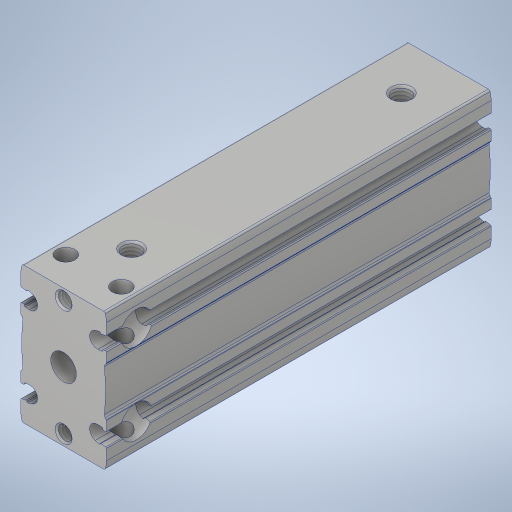
# Autodesk Inventor part: 4186566 DPDM-50---(h)
Saved by Autodesk Inventor 2024 (Build 280153000, 153)
## iProperties
Created: 2024-04-11
Part Number: 4186566 DPDM-50---(h)
Material: Aluminum 6061
Catalog Web Link: www.cadenas.de
Description: DPDM(h)-housing
Vendor: FESTO
Document SubType Name: Modeling
Designer: psAdmin
Manufacturer: FESTO
Mass: 104.929 g
Surface Area: 178.452 cm^2
Volume: 38.8626 cm^3
Density: 2.7 g/cm^3
Appearance: Aluminum - Flat
Category: PARTsolutions
Company: FESTO
PSOL_IDENT_0: {$CADENAS_DATA/23d-libs/festo/parts/d/dpdm/parts/dpdm_housing.prj},201 {VTYP=3D},{NB=4186566 DPDM-50
PSOL_IDENT_1: ---(h)},{LINA=4186566 DPDM-50---(h)},{NN=DPDM(h)},{DATE=23.02.2024 06:49:52},{GEOMDATE=23.02.2024 06
PSOL_IDENT_2: :49:00},{VERSION=},{LINEID=30},{WBVAR=VER,HUB,FUN,KOT},{WBNUMERIC=HUB}  {NB=4186566 DPDM-50---(h)},{
PSOL_IDENT_3: LINA=4186566 DPDM-50---(h)},{KT=DUMMY},{TNR=4186566},{TYP=DPDM},{VER=-},{VERNB=},{KOL=16},{HUB=50},{
PSOL_IDENT_4: HUB1=5,10,15,20,25,30,40,50},{FUN=-},{FUN1='-'},{FUNNB=},{KOT=-},{KOT1='-','H','T'},{KOTNB=},{MM=6.0
PSOL_IDENT_5: 00},{L2=40.000},{EE=M5},{EEN=5.000},{ET=4.500},{BG=6.000},{RT=M4},{RTN=4.000},{H2=19.000},{E=20.000}
PSOL_IDENT_6: ,{UO=32.000},{TO=27.000},{H3=13.000},{LX=7.000},{PL=24.100},{PR=11.000},{U1=0.000},{D5=4.300},{D6=7.
PSOL_IDENT_7: 500},{T1=6.000},{A1X=6.000},{A1Y=2.000},{A2X=6.100},{A2Y=9.100},{W2=10.000},{R1=47.500},{A3=11.500},
PSOL_IDENT_8: {L1=22.6},{L3=7.000},{DQ=4.000}
NB: 4186566 DPDM-50---(h)
NN: DPDM(h)
NT: housing
NBSYN: $TNR. $TYP.$VERNB.-$HUB.$FUNNB.$KOTNB.---(h)
LINA: 4186566 DPDM-50---(h)
CATALOG: Festo
TNR: 4186566
TYP: DPDM
VER: -
KOL: 16
HUB: 50
FUN: -
KOT: -
MM: 6
L2: 40
EE: M5
EEN: 5
ET: 4.5
BG: 6
RT: M4
RTN: 4
H2: 19
E: 20
UO: 32
TO: 27
H3: 13
LX: 7
PL: 24.1
PR: 11
U1: 0
D5: 4.3
D6: 7.5
T1: 6
A1X: 6
A1Y: 2
A2X: 6.1
A2Y: 9.1
W2: 10
R1: 47.5
A3: 11.5
L3: 7
DQ: 4
SUPPLIER: FESTO
ARTICLENO: 4186566 DPDM-50---(h)
BOMINFO: 4186566 DPDM-50---(h)
CREATOR: CADENAS GmbH
Title: 4186566 DPDM-50---(h)
Author: Cadenas PARTsolutions
Comments: housing
Autodesk Inventor part; units mm, degrees
sketch "Sketch_1" plane through (0, 0, 0) normal (0, 0, 1) x (1, 0, 0)
  line L0 (-10, -16) -> (10, -16)
  line L1 (10, -16) -> (10, 16)
  line L2 (10, 16) -> (-10, 16)
  line L3 (-10, 16) -> (-10, -16)
  constraints: 8 end point
extrude "Extrusion1" add sketch "Sketch_1" against normal blind 90
sketch "Sketch_2" plane through (0, 0, 0) normal (0, 0, 1) x (1, 0, 0)
  line L0 (-20, -26) -> (20, -26)
  line L1 (20, -26) -> (20, 26)
  line L2 (20, 26) -> (-20, 26)
  line L3 (-20, 26) -> (-20, -26)
  line L4 (-10, 8.0262) -> (-10, -8.0262)
  arc A0 (-10, -8.0262) -> (-9.7653, -8.2231) centre (-9.8, -8.0262) ccw
  line L5 (-9.7653, -8.2231) -> (-9.2952, -8.1403)
  arc A1 (-9.2952, -8.1403) -> (-9.1492, -7.9314) centre (-9.3265, -7.963) ccw
  arc A2 (-8.9688, -7.697) -> (-9.1492, -7.9314) centre (-8.9523, -7.8963) ccw
  line L6 (-8.9688, -7.697) -> (-8.0209, -7.6187)
  arc A3 (-7.3984, -11.149) -> (-8.0209, -7.6187) centre (-7.8727, -9.4126) ccw
  line L7 (-7.3984, -11.149) -> (-8.316, -11.3996)
  arc A4 (-8.5657, -11.241) -> (-8.316, -11.3996) centre (-8.3687, -11.2066) ccw
  arc A5 (-8.5657, -11.241) -> (-8.7743, -11.0947) centre (-8.743, -11.2719) ccw
  line L8 (-8.7743, -11.0947) -> (-9.8347, -11.2817)
  arc A6 (-9.8347, -11.2817) -> (-10, -11.4786) centre (-9.8, -11.4786) ccw
  line L9 (-10, -11.4786) -> (-10, -14)
  arc A7 (-10, -14) -> (-9.7564, -15.6923) centre (-4, -14) ccw
  arc A8 (-9.7564, -15.6923) -> (-9.3452, -16) centre (-9.3452, -15.5714) ccw
  line L10 (-9.3452, -16) -> (9.3452, -16)
  arc A9 (9.3452, -16) -> (9.7564, -15.6923) centre (9.3452, -15.5714) ccw
  arc A10 (9.7564, -15.6923) -> (10, -14) centre (4, -14) ccw
  line L11 (10, -14) -> (10, -11.4786)
  arc A11 (10, -11.4786) -> (9.8347, -11.2817) centre (9.8, -11.4786) ccw
  line L12 (9.8347, -11.2817) -> (8.7743, -11.0947)
  arc A12 (8.7743, -11.0947) -> (8.5657, -11.241) centre (8.743, -11.2719) ccw
  arc A13 (8.316, -11.3996) -> (8.5657, -11.241) centre (8.3687, -11.2066) ccw
  line L13 (8.316, -11.3996) -> (7.3984, -11.149)
  arc A14 (8.0209, -7.6187) -> (7.3984, -11.149) centre (7.8727, -9.4126) ccw
  line L14 (8.0209, -7.6187) -> (8.9688, -7.697)
  arc A15 (9.1492, -7.9314) -> (8.9688, -7.697) centre (8.9523, -7.8963) ccw
  arc A16 (9.1492, -7.9314) -> (9.2952, -8.1403) centre (9.3265, -7.963) ccw
  line L15 (9.2952, -8.1403) -> (9.7653, -8.2231)
  arc A17 (9.7653, -8.2231) -> (10, -8.0262) centre (9.8, -8.0262) ccw
  line L16 (10, -8.0262) -> (10, 8.0262)
  arc A18 (10, 8.0262) -> (9.7653, 8.2231) centre (9.8, 8.0262) ccw
  line L17 (9.7653, 8.2231) -> (9.2952, 8.1403)
  arc A19 (9.2952, 8.1403) -> (9.1492, 7.9314) centre (9.3265, 7.963) ccw
  arc A20 (8.9688, 7.697) -> (9.1492, 7.9314) centre (8.9523, 7.8963) ccw
  line L18 (8.9688, 7.697) -> (8.0209, 7.6187)
  arc A21 (7.3984, 11.149) -> (8.0209, 7.6187) centre (7.8727, 9.4126) ccw
  line L19 (7.3984, 11.149) -> (8.316, 11.3996)
  arc A22 (8.5657, 11.241) -> (8.316, 11.3996) centre (8.3687, 11.2066) ccw
  arc A23 (8.5657, 11.241) -> (8.7743, 11.0947) centre (8.743, 11.2719) ccw
  line L20 (8.7743, 11.0947) -> (9.8347, 11.2817)
  arc A24 (9.8347, 11.2817) -> (10, 11.4786) centre (9.8, 11.4786) ccw
  line L21 (10, 11.4786) -> (10, 14)
  arc A25 (10, 14) -> (9.7564, 15.6923) centre (4, 14) ccw
  arc A26 (9.7564, 15.6923) -> (9.3452, 16) centre (9.3452, 15.5714) ccw
  line L22 (9.3452, 16) -> (-9.3452, 16)
  arc A27 (-9.3452, 16) -> (-9.7564, 15.6923) centre (-9.3452, 15.5714) ccw
  arc A28 (-9.7564, 15.6923) -> (-10, 14) centre (-4, 14) ccw
  line L23 (-10, 14) -> (-10, 11.4786)
  arc A29 (-10, 11.4786) -> (-9.8347, 11.2817) centre (-9.8, 11.4786) ccw
  line L24 (-9.8347, 11.2817) -> (-8.7743, 11.0947)
  arc A30 (-8.7743, 11.0947) -> (-8.5657, 11.241) centre (-8.743, 11.2719) ccw
  arc A31 (-8.316, 11.3996) -> (-8.5657, 11.241) centre (-8.3687, 11.2066) ccw
  line L25 (-8.316, 11.3996) -> (-7.3984, 11.149)
  arc A32 (-8.0209, 7.6187) -> (-7.3984, 11.149) centre (-7.8727, 9.4126) ccw
  line L26 (-8.0209, 7.6187) -> (-8.9688, 7.697)
  arc A33 (-9.1492, 7.9314) -> (-8.9688, 7.697) centre (-8.9523, 7.8963) ccw
  arc A34 (-9.1492, 7.9314) -> (-9.2952, 8.1403) centre (-9.3265, 7.963) ccw
  line L27 (-9.2952, 8.1403) -> (-9.7653, 8.2231)
  arc A35 (-9.7653, 8.2231) -> (-10, 8.0262) centre (-9.8, 8.0262) ccw
  constraints: 72 point on circle, 56 end point, 36 centre point
extrude "Extrusion2" cut sketch "Sketch_2" against normal blind 90
sketch "Sketch_3" plane through (0, 0, 0) normal (0, 0, 1) x (1, 0, 0)
  line L0 (-15, -21) -> (15, -21)
  line L1 (15, -21) -> (15, 21)
  line L2 (15, 21) -> (-15, 21)
  line L3 (-15, 21) -> (-15, -21)
  arc A0 (-10, 5.8228) -> (-9.9532, 5.6942) centre (-9.8, 5.8228) ccw
  line L4 (-9.9532, 5.6942) -> (-9.7222, 5.419)
  arc A1 (-9.5507, 4.8601) -> (-9.7222, 5.419) centre (-10.2968, 4.9369) ccw
  arc A2 (-9.5507, 4.8601) -> (-9.5507, -4.8601) centre (37.7, 0) ccw
  arc A3 (-9.7222, -5.419) -> (-9.5507, -4.8601) centre (-10.2968, -4.9369) ccw
  line L5 (-9.7222, -5.419) -> (-9.9532, -5.6942)
  arc A4 (-9.9532, -5.6942) -> (-10, -5.8228) centre (-9.8, -5.8228) ccw
  line L6 (-10, -5.8228) -> (-10, -16)
  line L7 (-10, -16) -> (10, -16)
  line L8 (10, -16) -> (10, -5.8228)
  arc A5 (10, -5.8228) -> (9.9532, -5.6942) centre (9.8, -5.8228) ccw
  line L9 (9.9532, -5.6942) -> (9.7222, -5.419)
  arc A6 (9.5507, -4.8601) -> (9.7222, -5.419) centre (10.2968, -4.9369) ccw
  arc A7 (9.5507, -4.8601) -> (9.5507, 4.8601) centre (-37.7, 0) ccw
  arc A8 (9.7222, 5.419) -> (9.5507, 4.8601) centre (10.2968, 4.9369) ccw
  line L10 (9.7222, 5.419) -> (9.9532, 5.6942)
  arc A9 (9.9532, 5.6942) -> (10, 5.8228) centre (9.8, 5.8228) ccw
  line L11 (10, 5.8228) -> (10, 16)
  line L12 (10, 16) -> (-10, 16)
  line L13 (-10, 16) -> (-10, 5.8228)
  constraints: 28 end point, 20 point on circle, 10 centre point
extrude "Extrusion3" cut sketch "Sketch_3" against normal blind 90
sketch "Sketch_6" plane through (0, 0, 0) normal (1, 0, 0) x (0, 1, 0)
  line L0 (0, -72.4) -> (0, 0)
  line L1 (0, 0) -> (3, 0)
  line L2 (3, 0) -> (3, -17.4)
  line L3 (3, -17.4) -> (8, -17.4)
  line L4 (8, -17.4) -> (8, -72.4)
  line L5 (8, -72.4) -> (0, -72.4)
  line L6 (0, -72.4) -> (0, 0)
  constraints: 14 end point
revolve "Revolution1" cut sketch "Sketch_6" angle 360 about axis through (0, 0, -72.4) along (0, 0, -1)
sketch "Sketch_8" plane through (0, 0, 0) normal (1, 0, 0) x (0, 1, 0)
  line L0 (0, -90) -> (0, -87.9)
  line L1 (9, -87.9) -> (7, -87.9)
  line L2 (7, -87.9) -> (7, -89.7)
  line L3 (7, -89.7) -> (6.7, -90)
  line L4 (6.7, -90) -> (9.4, -90)
  line L5 (9.4, -90) -> (9, -89.6)
  line L6 (9, -89.6) -> (9, -87.9)
  constraints: 14 end point
revolve "Revolution2" cut sketch "Sketch_8" angle 360 about axis through (0, 0, -90) along (0, 0, -1)
sketch "Sketch6" plane through (-9.3452, 16, -90) normal (0, 1, 0) x (1, 0, 0)
  point P0 (9.3452, -74.1)
hole "Hole1" at (0, 16, -15.9) direction (0, -1, 0) diameter 4.134 depth 6 countersink diameter 5 countersink angle 90 thread size "M5x0.8" class "6H" standard "ISO Metric profile"
pattern_linear "Rectangular Pattern1" count 2 spacing 63.1 along (0, 0, -1) of "Hole1"
sketch "Sketch7" plane through (0, 0, -90) normal (0, 0, -1) x (-1, 0, 0)
  point P0 (0, 13.5)
hole "Hole2" at (0, 13.5, -90) direction (0, 0, 1) diameter 3.242 depth 7.5 countersink diameter 4 countersink angle 90 thread size "M4x0.7" class "6H" standard "ISO Metric profile"
pattern_linear "Rectangular Pattern2" count 2 spacing 27 along (0, -1, 0) of "Hole2"
sketch "Sketch8" plane through (0, 0, 0) normal (0, 0, 1) x (1, 0, 0)
  point P0 (0, 13.5)
hole "Hole3" at (0, 13.5, 0) direction (0, 0, -1) diameter 3.242 depth 7.5 countersink diameter 4 countersink angle 90 thread size "M4x0.7" class "6H" standard "ISO Metric profile"
sketch "Sketch9" plane through (0, 0, 0) normal (0, 0, 1) x (1, 0, 0)
  point P0 (0, -13.5)
hole "Hole4" at (0, -13.5, 0) direction (0, 0, -1) diameter 3.242 depth 7.5 countersink diameter 4 countersink angle 90 thread size "M4x0.7" class "6H" standard "ISO Metric profile"
sketch "Sketch10" plane through (-9.3452, -16, 0) normal (0, -1, 0) x (1, 0, 0)
  point P0 (15.8452, -7)
hole "Hole5" at (6.5, -16, -7) direction (0, 1, 0) diameter 4.3 depth 32
pattern_linear "Rectangular Pattern3" count 2 spacing 13 along (-1, 0, 0) of "Hole5"
sketch "Sketch_28" plane through (0, 0, -7) normal (0, 0, 1) x (1, 0, 0)
  line L0 (10, 9.5) -> (-10, 9.5)
  line L1 (-10, 9.5) -> (-10, 13.25)
  line L2 (-10, 13.25) -> (-4, 13.25)
  line L3 (-4, 13.25) -> (-4, 11.65)
  line L4 (-4, 11.65) -> (4, 11.65)
  line L5 (4, 11.65) -> (4, 13.25)
  line L6 (4, 13.25) -> (10, 13.25)
  line L7 (10, 13.25) -> (10, 9.5)
  line L8 (10, 9.5) -> (-10, 9.5)
  constraints: 18 end point
revolve "Revolution3" cut sketch "Sketch_28" angle 360 about axis through (10, 9.5, -7) along (1, 0, 0)
pattern_linear "Rectangular Pattern4" count 2 spacing 19 along (0, -1, 0) of "Revolution3"
ref_plane "ANBAU_XY" through (0, 0, 0) normal (0, 0, 1) x (1, 0, 0)
ref_plane "ANBAU_YZ" through (0, 0, 0) normal (1, 0, 0) x (0, 1, 0)
ref_plane "ANBAU_ZX" through (0, 0, 0) normal (0, 1, 0) x (0, 0, 1)
ref_plane "CP_DR_XY" through (0, 16, -79) normal (0, -1, 0) x (1, 0, 0)
ref_plane "CP_DR_YZ" through (0, 16, -79) normal (1, 0, 0) x (0, 0, 1)
ref_plane "CP_DR_ZX" through (0, 16, -79) normal (0, 0, 1) x (0, -1, 0)
ref_plane "CP_ROD1_XY" through (0, 0, -72.4) normal (0, 0, 1) x (1, 0, 0)
ref_plane "CP_ROD1_YZ" through (0, 0, -72.4) normal (1, 0, 0) x (0, 1, 0)
ref_plane "CP_ROD1_ZX" through (0, 0, -72.4) normal (0, 1, 0) x (0, 0, 1)
ref_plane "CP_ROD_P_XY" through (0, 0, -72.4) normal (0, 0, -1) x (1, 0, 0)
ref_plane "CP_ROD_P_YZ" through (0, 0, -72.4) normal (1, 0, 0) x (0, -1, 0)
ref_plane "CP_ROD_P_ZX" through (0, 0, -72.4) normal (0, -1, 0) x (0, 0, -1)
ref_plane "SCHRAUBE_1_XY" through (4, 9.5, -7) normal (-1, 0, 0) x (0, 0, -1)
ref_plane "SCHRAUBE_1_YZ" through (4, 9.5, -7) normal (0, 0, -1) x (0, -1, 0)
ref_plane "SCHRAUBE_1_ZX" through (4, 9.5, -7) normal (0, -1, 0) x (-1, 0, 0)
ref_plane "SCHRAUBE_2_XY" through (4, -9.5, -7) normal (-1, 0, 0) x (0, 0, -1)
ref_plane "SCHRAUBE_2_YZ" through (4, -9.5, -7) normal (0, 0, -1) x (0, -1, 0)
ref_plane "SCHRAUBE_2_ZX" through (4, -9.5, -7) normal (0, -1, 0) x (-1, 0, 0)
ref_plane "SCHRAUBE_B_1_XY" through (6.5, 16, -7) normal (0, -1, 0) x (1, 0, 0)
ref_plane "SCHRAUBE_B_1_YZ" through (6.5, 16, -7) normal (1, 0, 0) x (0, 0, 1)
ref_plane "SCHRAUBE_B_1_ZX" through (6.5, 16, -7) normal (0, 0, 1) x (0, -1, 0)
ref_plane "SCHRAUBE_B_2_XY" through (-6.5, 16, -7) normal (0, -1, 0) x (1, 0, 0)
ref_plane "SCHRAUBE_B_2_YZ" through (-6.5, 16, -7) normal (1, 0, 0) x (0, 0, 1)
ref_plane "SCHRAUBE_B_2_ZX" through (-6.5, 16, -7) normal (0, 0, 1) x (0, -1, 0)
ref_plane "TO_HALTER_XY" through (0, -16, -7) normal (0, 1, 0) x (1, 0, 0)
ref_plane "TO_HALTER_YZ" through (0, -16, -7) normal (1, 0, 0) x (0, 0, -1)
ref_plane "TO_HALTER_ZX" through (0, -16, -7) normal (0, 0, -1) x (0, 1, 0)
ref_plane "TO_QSML_1_XY" through (0, 16, -15.9) normal (0, -1, 0) x (0, 0, -1)
ref_plane "TO_QSML_1_YZ" through (0, 16, -15.9) normal (0, 0, -1) x (1, 0, 0)
ref_plane "TO_QSML_1_ZX" through (0, 16, -15.9) normal (1, 0, 0) x (0, -1, 0)
ref_plane "TO_QSML_2_XY" through (0, 16, -79) normal (0, -1, 0) x (0, 0, -1)
ref_plane "TO_QSML_2_YZ" through (0, 16, -79) normal (0, 0, -1) x (1, 0, 0)
ref_plane "TO_QSML_2_ZX" through (0, 16, -79) normal (1, 0, 0) x (0, -1, 0)
body "Solid1"
